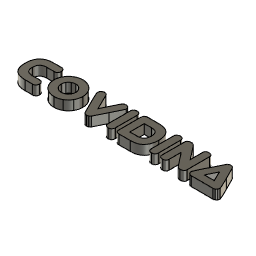
covidina - letras v1 (Autodesk Fusion 360 design; units mm, degrees)
Autodesk Fusion 360 part; units mm, degrees
sketch "Sketch1" plane through (0, 0, 0) normal (0, 0, 1) x (1, 0, 0)
  line L0 (19.5265, 28.0047) -> (21.0645, 28.0008)
  spline S0 degree 3 poles (21.0645, 28.0008) (21.574, 27.993) (21.8306, 27.7392) (21.8336, 27.2396) knots 0 0 0 0 1 1 1 1
  spline S1 degree 3 poles (21.8336, 27.2396) (21.8306, 26.7213) (21.573, 26.4637) (21.0606, 26.4666) knots 0 0 0 0 1 1 1 1
  line L1 (21.0606, 26.4666) -> (19.5304, 26.4627)
  spline S2 degree 3 poles (19.5304, 26.4627) (18.5076, 26.4705) (17.9962, 25.9601) (17.9962, 24.9325) knots 0 0 0 0 1 1 1 1
  spline S3 degree 3 poles (17.9962, 24.9325) (17.9962, 23.9116) (18.5076, 23.3993) (19.5304, 23.3944) knots 0 0 0 0 1 1 1 1
  line L2 (19.5304, 23.3944) -> (21.0606, 23.3944)
  spline S4 degree 3 poles (21.0606, 23.3944) (21.573, 23.3837) (21.8297, 23.1299) (21.8297, 22.6332) knots 0 0 0 0 1 1 1 1
  spline S5 degree 3 poles (21.8297, 22.6332) (21.8297, 22.1198) (21.5759, 21.8622) (21.0684, 21.8602) knots 0 0 0 0 1 1 1 1
  line L3 (21.0684, 21.8602) -> (19.5304, 21.8602)
  spline S6 degree 3 poles (19.5304, 21.8602) (17.4819, 21.8602) (16.4562, 22.885) (16.4542, 24.9364) knots 0 0 0 0 1 1 1 1
  spline S7 degree 3 poles (16.4542, 24.9364) (16.4542, 26.9839) (17.478, 28.0067) (19.5265, 28.0047) knots 0 0 0 0 1 1 1 1
  spline S8 degree 3 poles (25.671, 28.0047) (26.1863, 28.0047) (26.6879, 27.872) (27.1778, 27.6065) knots 0 0 0 0 1 1 1 1
  spline S9 degree 3 poles (27.1778, 27.6065) (27.6697, 27.3411) (28.0542, 26.9605) (28.3333, 26.4666) knots 0 0 0 0 1 1 1 1
  spline S10 degree 3 poles (28.3333, 26.4666) (28.6115, 25.9748) (28.751, 25.4614) (28.751, 24.9286) knots 0 0 0 0 1 1 1 1
  spline S11 degree 3 poles (28.751, 24.9286) (28.751, 24.3947) (28.6154, 23.8833) (28.345, 23.3944) knots 0 0 0 0 1 1 1 1
  spline S12 degree 3 poles (28.345, 23.3944) (28.0737, 22.9074) (27.6941, 22.5287) (27.2052, 22.2584) knots 0 0 0 0 1 1 1 1
  spline S13 degree 3 poles (27.2052, 22.2584) (26.7152, 21.9871) (26.2038, 21.8524) (25.671, 21.8524) knots 0 0 0 0 1 1 1 1
  spline S14 degree 3 poles (25.671, 21.8524) (25.1401, 21.8524) (24.6297, 21.9871) (24.1407, 22.2584) knots 0 0 0 0 1 1 1 1
  spline S15 degree 3 poles (24.1407, 22.2584) (23.6508, 22.5287) (23.2712, 22.9074) (23.0008, 23.3944) knots 0 0 0 0 1 1 1 1
  spline S16 degree 3 poles (23.0008, 23.3944) (22.7295, 23.8833) (22.5949, 24.3947) (22.5949, 24.9286) knots 0 0 0 0 1 1 1 1
  spline S17 degree 3 poles (22.5949, 24.9286) (22.5949, 25.4614) (22.7315, 25.9748) (23.0047, 26.4666) knots 0 0 0 0 1 1 1 1
  spline S18 degree 3 poles (23.0047, 26.4666) (23.28, 26.9605) (23.6625, 27.3411) (24.1524, 27.6065) knots 0 0 0 0 1 1 1 1
  spline S19 degree 3 poles (24.1524, 27.6065) (24.6443, 27.872) (25.1498, 28.0047) (25.671, 28.0047) knots 0 0 0 0 1 1 1 1
  spline S20 degree 3 poles (25.6749, 26.4744) (25.4143, 26.4744) (25.1616, 26.4081) (24.9176, 26.2753) knots 0 0 0 0 1 1 1 1
  spline S21 degree 3 poles (24.9176, 26.2753) (24.6726, 26.1446) (24.4813, 25.9562) (24.3437, 25.7093) knots 0 0 0 0 1 1 1 1
  spline S22 degree 3 poles (24.3437, 25.7093) (24.2051, 25.4614) (24.1368, 25.2038) (24.1368, 24.9364) knots 0 0 0 0 1 1 1 1
  spline S23 degree 3 poles (24.1368, 24.9364) (24.1368, 24.668) (24.2042, 24.4113) (24.3398, 24.1673) knots 0 0 0 0 1 1 1 1
  spline S24 degree 3 poles (24.3398, 24.1673) (24.4745, 23.9253) (24.6648, 23.736) (24.9098, 23.6013) knots 0 0 0 0 1 1 1 1
  spline S25 degree 3 poles (24.9098, 23.6013) (25.1537, 23.4656) (25.4094, 23.3983) (25.6749, 23.3983) knots 0 0 0 0 1 1 1 1
  spline S26 degree 3 poles (25.6749, 23.3983) (25.9423, 23.3983) (26.199, 23.4656) (26.4439, 23.6013) knots 0 0 0 0 1 1 1 1
  spline S27 degree 3 poles (26.4439, 23.6013) (26.6879, 23.736) (26.8782, 23.9253) (27.0139, 24.1673) knots 0 0 0 0 1 1 1 1
  spline S28 degree 3 poles (27.0139, 24.1673) (27.1485, 24.4113) (27.2169, 24.668) (27.2169, 24.9364) knots 0 0 0 0 1 1 1 1
  spline S29 degree 3 poles (27.2169, 24.9364) (27.2169, 25.2038) (27.1476, 25.4614) (27.01, 25.7093) knots 0 0 0 0 1 1 1 1
  spline S30 degree 3 poles (27.01, 25.7093) (26.8714, 25.9562) (26.6791, 26.1446) (26.4322, 26.2753) knots 0 0 0 0 1 1 1 1
  spline S31 degree 3 poles (26.4322, 26.2753) (26.1873, 26.4081) (25.9345, 26.4744) (25.6749, 26.4744) knots 0 0 0 0 1 1 1 1
  spline S32 degree 3 poles (34.8988, 28.0125) (35.0257, 28.0125) (35.1506, 27.9784) (35.2736, 27.911) knots 0 0 0 0 1 1 1 1
  spline S33 degree 3 poles (35.2736, 27.911) (35.3985, 27.8456) (35.4942, 27.751) (35.5625, 27.626) knots 0 0 0 0 1 1 1 1
  spline S34 degree 3 poles (35.5625, 27.626) (35.6327, 27.5031) (35.6679, 27.3762) (35.6679, 27.2435) knots 0 0 0 0 1 1 1 1
  spline S35 degree 3 poles (35.6679, 27.2435) (35.6679, 27.1107) (35.2824, 26.2734) (34.5124, 24.7334) knots 0 0 0 0 1 1 1 1
  spline S36 degree 3 poles (34.5124, 24.7334) (33.7414, 23.1924) (33.3227, 22.3609) (33.2554, 22.2389) knots 0 0 0 0 1 1 1 1
  spline S37 degree 3 poles (33.2554, 22.2389) (33.1871, 22.1189) (33.0924, 22.0252) (32.9704, 21.9578) knots 0 0 0 0 1 1 1 1
  spline S38 degree 3 poles (32.9704, 21.9578) (32.8504, 21.8895) (32.7245, 21.8563) (32.5917, 21.8563) knots 0 0 0 0 1 1 1 1
  spline S39 degree 3 poles (32.5917, 21.8563) (32.4561, 21.8563) (32.3273, 21.8895) (32.2053, 21.9578) knots 0 0 0 0 1 1 1 1
  spline S40 degree 3 poles (32.2053, 21.9578) (32.0823, 22.0252) (31.9876, 22.1189) (31.9203, 22.2389) knots 0 0 0 0 1 1 1 1
  spline S41 degree 3 poles (31.9203, 22.2389) (31.8549, 22.3609) (31.4382, 23.1924) (30.6711, 24.7334) knots 0 0 0 0 1 1 1 1
  spline S42 degree 3 poles (30.6711, 24.7334) (29.906, 26.2734) (29.5234, 27.1107) (29.5234, 27.2435) knots 0 0 0 0 1 1 1 1
  spline S43 degree 3 poles (29.5234, 27.2435) (29.5234, 27.3762) (29.5566, 27.5031) (29.6249, 27.626) knots 0 0 0 0 1 1 1 1
  spline S44 degree 3 poles (29.6249, 27.626) (29.6952, 27.751) (29.7908, 27.8456) (29.9138, 27.911) knots 0 0 0 0 1 1 1 1
  spline S45 degree 3 poles (29.9138, 27.911) (30.0358, 27.9784) (30.1617, 28.0125) (30.2925, 28.0125) knots 0 0 0 0 1 1 1 1
  spline S46 degree 3 poles (30.2925, 28.0125) (30.4193, 28.0125) (30.5442, 27.9784) (30.6672, 27.911) knots 0 0 0 0 1 1 1 1
  spline S47 degree 3 poles (30.6672, 27.911) (30.7921, 27.8456) (30.8878, 27.751) (30.9561, 27.626) knots 0 0 0 0 1 1 1 1
  spline S48 degree 3 poles (30.9561, 27.626) (31.0264, 27.5031) (31.5709, 26.3934) (32.5917, 24.2962) knots 0 0 0 0 1 1 1 1
  spline S49 degree 3 poles (32.5917, 24.2962) (33.6165, 26.3934) (34.163, 27.5031) (34.2313, 27.626) knots 0 0 0 0 1 1 1 1
  spline S50 degree 3 poles (34.2313, 27.626) (34.3016, 27.751) (34.3972, 27.8456) (34.5202, 27.911) knots 0 0 0 0 1 1 1 1
  spline S51 degree 3 poles (34.5202, 27.911) (34.6422, 27.9784) (34.7681, 28.0125) (34.8988, 28.0125) knots 0 0 0 0 1 1 1 1
  spline S52 degree 3 poles (37.1977, 28.0047) (37.7101, 27.9988) (37.9707, 27.7451) (37.9785, 27.2435) knots 0 0 0 0 1 1 1 1
  line L4 (37.9785, 27.2435) -> (37.9785, 22.6254)
  spline S53 degree 3 poles (37.9785, 22.6254) (37.9726, 22.112) (37.715, 21.8524) (37.2055, 21.8446) knots 0 0 0 0 1 1 1 1
  spline S54 degree 3 poles (37.2055, 21.8446) (36.6922, 21.8554) (36.4365, 22.114) (36.4365, 22.6215) knots 0 0 0 0 1 1 1 1
  line L5 (36.4365, 22.6215) -> (36.4365, 27.2396)
  spline S55 degree 3 poles (36.4365, 27.2396) (36.4336, 27.7471) (36.6873, 28.0018) (37.1977, 28.0047) knots 0 0 0 0 1 1 1 1
  line L6 (39.4996, 28.0047) -> (41.8067, 28.0047)
  spline S56 degree 3 poles (41.8067, 28.0047) (43.8571, 28.0018) (44.8828, 26.978) (44.8828, 24.9325) knots 0 0 0 0 1 1 1 1
  spline S57 degree 3 poles (44.8828, 24.9325) (44.8799, 22.8889) (43.8805, 21.8651) (41.8848, 21.8602) knots 0 0 0 0 1 1 1 1
  line L7 (41.8848, 21.8602) -> (39.4996, 21.8602)
  spline S58 degree 3 poles (39.4996, 21.8602) (38.9862, 21.8554) (38.7305, 22.111) (38.7305, 22.6293) knots 0 0 0 0 1 1 1 1
  line L8 (38.7305, 22.6293) -> (38.7305, 27.2357)
  spline S59 degree 3 poles (38.7305, 27.2357) (38.7305, 27.7432) (38.9862, 27.9988) (39.4996, 28.0047) knots 0 0 0 0 1 1 1 1
  line L9 (40.2725, 26.4627) -> (40.2725, 23.4022)
  line L10 (40.2725, 23.4022) -> (41.8106, 23.4022)
  spline S60 degree 3 poles (41.8106, 23.4022) (42.8304, 23.3944) (43.3379, 23.9068) (43.333, 24.9403) knots 0 0 0 0 1 1 1 1
  spline S61 degree 3 poles (43.333, 24.9403) (43.3379, 25.9494) (42.8295, 26.4569) (41.8067, 26.4627) knots 0 0 0 0 1 1 1 1
  line L11 (41.8067, 26.4627) -> (40.2725, 26.4627)
  spline S62 degree 3 poles (46.4164, 28.0047) (46.9288, 27.9988) (47.1894, 27.7451) (47.1972, 27.2435) knots 0 0 0 0 1 1 1 1
  line L12 (47.1972, 27.2435) -> (47.1972, 22.6254)
  spline S63 degree 3 poles (47.1972, 22.6254) (47.1913, 22.112) (46.9337, 21.8524) (46.4242, 21.8446) knots 0 0 0 0 1 1 1 1
  spline S64 degree 3 poles (46.4242, 21.8446) (45.9109, 21.8554) (45.6552, 22.114) (45.6552, 22.6215) knots 0 0 0 0 1 1 1 1
  line L13 (45.6552, 22.6215) -> (45.6552, 27.2396)
  spline S65 degree 3 poles (45.6552, 27.2396) (45.6523, 27.7471) (45.906, 28.0018) (46.4164, 28.0047) knots 0 0 0 0 1 1 1 1
  spline S66 degree 3 poles (48.8198, 27.9969) (49.1009, 27.9754) (49.3243, 27.87) (49.4912, 27.6807) knots 0 0 0 0 1 1 1 1
  line L14 (49.4912, 27.6807) -> (51.7905, 24.7451)
  line L15 (51.7905, 24.7451) -> (51.7905, 27.3255)
  spline S67 degree 3 poles (51.7905, 27.3255) (51.8003, 27.7646) (52.0189, 27.9891) (52.4463, 27.9969) knots 0 0 0 0 1 1 1 1
  spline S68 degree 3 poles (52.4463, 27.9969) (53.0212, 27.9891) (53.311, 27.7597) (53.3169, 27.3098) knots 0 0 0 0 1 1 1 1
  line L16 (53.3169, 27.3098) -> (53.3247, 22.5278)
  spline S69 degree 3 poles (53.3247, 22.5278) (53.3188, 22.0876) (53.026, 21.8651) (52.4463, 21.8602) knots 0 0 0 0 1 1 1 1
  spline S70 degree 3 poles (52.4463, 21.8602) (52.1809, 21.8622) (51.9662, 21.9676) (51.8022, 22.1764) knots 0 0 0 0 1 1 1 1
  line L17 (51.8022, 22.1764) -> (49.4912, 25.1042)
  line L18 (49.4912, 25.1042) -> (49.4912, 22.5278)
  spline S71 degree 3 poles (49.4912, 22.5278) (49.4883, 22.0847) (49.2648, 21.8622) (48.8198, 21.8602) knots 0 0 0 0 1 1 1 1
  spline S72 degree 3 poles (48.8198, 21.8602) (48.242, 21.8583) (47.9512, 22.0827) (47.9493, 22.5356) knots 0 0 0 0 1 1 1 1
  line L19 (47.9493, 22.5356) -> (47.9493, 27.3294)
  spline S73 degree 3 poles (47.9493, 27.3294) (47.9463, 27.7715) (48.2362, 27.994) (48.8198, 27.9969) knots 0 0 0 0 1 1 1 1
  spline S74 degree 3 poles (54.8706, 21.8563) (54.7398, 21.8563) (54.6139, 21.8885) (54.4919, 21.9539) knots 0 0 0 0 1 1 1 1
  spline S75 degree 3 poles (54.4919, 21.9539) (54.3689, 22.0183) (54.2733, 22.112) (54.203, 22.235) knots 0 0 0 0 1 1 1 1
  spline S76 degree 3 poles (54.203, 22.235) (54.1347, 22.3599) (54.1015, 22.4897) (54.1015, 22.6254) knots 0 0 0 0 1 1 1 1
  spline S77 degree 3 poles (54.1015, 22.6254) (54.1015, 22.7581) (54.4841, 23.5935) (55.2492, 25.1316) knots 0 0 0 0 1 1 1 1
  spline S78 degree 3 poles (55.2492, 25.1316) (56.0163, 26.6716) (56.433, 27.5031) (56.4984, 27.626) knots 0 0 0 0 1 1 1 1
  spline S79 degree 3 poles (56.4984, 27.626) (56.5658, 27.748) (56.6604, 27.8427) (56.7834, 27.911) knots 0 0 0 0 1 1 1 1
  spline S80 degree 3 poles (56.7834, 27.911) (56.9054, 27.9784) (57.0342, 28.0125) (57.1699, 28.0125) knots 0 0 0 0 1 1 1 1
  spline S81 degree 3 poles (57.1699, 28.0125) (57.3026, 28.0125) (57.4285, 27.9784) (57.5485, 27.911) knots 0 0 0 0 1 1 1 1
  spline S82 degree 3 poles (57.5485, 27.911) (57.6705, 27.8427) (57.7652, 27.748) (57.8335, 27.626) knots 0 0 0 0 1 1 1 1
  spline S83 degree 3 poles (57.8335, 27.626) (57.9008, 27.5031) (58.3195, 26.6716) (59.0905, 25.1316) knots 0 0 0 0 1 1 1 1
  spline S84 degree 3 poles (59.0905, 25.1316) (59.8605, 23.5935) (60.246, 22.7581) (60.246, 22.6254) knots 0 0 0 0 1 1 1 1
  spline S85 degree 3 poles (60.246, 22.6254) (60.246, 22.4897) (60.2109, 22.3599) (60.1406, 22.235) knots 0 0 0 0 1 1 1 1
  spline S86 degree 3 poles (60.1406, 22.235) (60.0723, 22.112) (59.9766, 22.0183) (59.8517, 21.9539) knots 0 0 0 0 1 1 1 1
  spline S87 degree 3 poles (59.8517, 21.9539) (59.7287, 21.8885) (59.6038, 21.8563) (59.477, 21.8563) knots 0 0 0 0 1 1 1 1
  line L20 (59.477, 21.8563) -> (54.8706, 21.8563)
  line L21 (58.22, 23.4061) -> (57.1699, 25.5688)
  line L22 (57.1699, 25.5688) -> (56.1119, 23.4061)
  line L23 (56.1119, 23.4061) -> (58.22, 23.4061)
extrude "Extrude1" add sketch "Sketch1" along normal blind 2 makes body 1 at (45.6552, 24.1608, 0.6667) makes body 2 at (27.9912, 26.0072, 0) makes body 3 at (31.4063, 25.5519, 0) makes body 4 at (48.4632, 24.9897, 0) makes body 5 at (39.2445, 24.4224, 0) makes body 6 at (20.5531, 22.3716, 0) makes body 7 at (36.4365, 24.1608, 0.6667) makes body 8 at (57.5225, 22.3729, 0)
